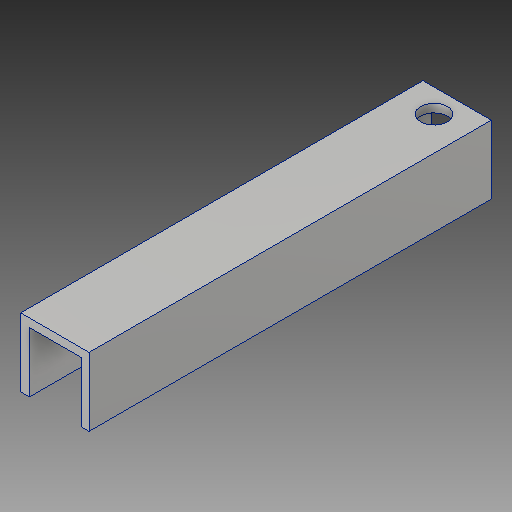
# Autodesk Inventor part: ㄇ形件
Saved by Autodesk Inventor 2017 (Build 210142000, 142)
## iProperties
Part Number: ㄇ形件
Material: 鋁合金 6061
Document SubType Name: Modeling
Designer: user
Density: 2.7 g/cm^3
Appearance: 鋁 - 平面
Author: user
Autodesk Inventor part; units mm, degrees
ref_plane "YZ Plane" through (0, 0, 0) normal (1, 0, 0) x (0, 1, 0)
ref_plane "XZ Plane" through (0, 0, 0) normal (0, 1, 0) x (-1, 0, 0)
ref_plane "XY Plane" through (0, 0, 0) normal (0, 0, 1) x (1, 0, 0)
sketch "草圖1" plane through (0, 0, 0) normal (0, 0, 1) x (1, 0, 0)
  line L0 (0, 0) -> (0, 25.5)
  line L1 (0, 25.5) -> (25.5, 25.5)
  line L2 (25.5, 25.5) -> (25.5, 0)
  line L3 (25.5, 0) -> (0, 0)
  dimension "d0" = 25.5
  dimension "d1" = 25.5
  constraints: 8 end point, 3 perpendicular, 1 vertical
  measures "d0" distance of L0.end L1.end
  measures "d1" distance of L0.start L0.end
extrude "擠出1" add sketch "草圖1" along normal blind 150
sketch "草圖2" plane through (0, 0, 150) normal (0, 0, 1) x (1, 0, 0)
  line L0 (3.28, -7.124) -> (22.5, -7.124)
  line L1 (22.5, -7.124) -> (22.5, 22.4)
  line L2 (22.5, 22.4) -> (3.28, 22.4)
  line L3 (3.28, 22.4) -> (3.28, -7.124)
  line L4 (0, 0) -> (25.5, 0) projected
  dimension "d4" = 19.22
  dimension "d5" = 22.4
  dimension "d6" = 3
  constraints: 8 end point, 2 parallel, 1 horizontal, 1 perpendicular
  measures "d4" distance of L1.end L2.end
  measures "d5" distance between parallel lines of L4 L2
  measures "d6" distance from line of L4.end L1
extrude "擠出2" cut sketch "草圖2" against normal through all
sketch "草圖3" plane through (3.28, 22.4, 150) normal (0, -1, 0) x (1, 0, 0)
  circle A0 centre (9.61, -141.2584) radius 5
  point P0 (-3.28, -150)
  dimension "d9" = 10
  constraints: 1 centre point
  measures "d9" diameter of A0
extrude "擠出3" cut sketch "草圖3" against normal blind 150
